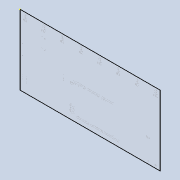
# Autodesk Inventor part: MAIN CNTRL_v02 Bottom
Saved by Autodesk Inventor 2022 (Build 260153000, 153)
## iProperties
Created: 2023-03-29
Part Number: MAIN CNTRL_v02 Bottom
Material: Generic
Document SubType Name: Modeling
Designer: SB13FLLT004
Density: 1 g/cm^3
Appearance: Clear - Light
Author: SB13FLLT004
Autodesk Inventor part; units mm, degrees
ref_plane "YZ Plane" through (0, 0, 0) normal (1, 0, 0) x (0, 1, 0)
ref_plane "XZ Plane" through (0, 0, 0) normal (0, 1, 0) x (-1, 0, 0)
ref_plane "XY Plane" through (0, 0, 0) normal (0, 0, 1) x (1, 0, 0)
sketch "Sketch1" plane through (0, 0, 0) normal (0, 0, 1) x (1, 0, 0)
  line L0 (0, 0) -> (228.6, 0)
  line L1 (228.6, 0) -> (228.6, -114.3)
  line L2 (228.6, -114.3) -> (0, -114.3)
  line L3 (0, -114.3) -> (0, 0)
  dimension "d8" = 228.6
  constraints: 1 coincident, 1 horizontal, 2 other
  measures "d8" distance of L0.start L0.end
extrude "Extrusion1" add sketch "Sketch1" along normal blind 0.254
body "Solid1"
